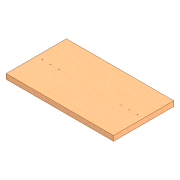
# Autodesk Inventor part: SGB-8-platform
Saved by Autodesk Inventor 2020 (Build 240168000, 168)
## iProperties
Created: 2021-06-24
Part Number: SGB-8-platform
Material: Generic
Document SubType Name: Modeling
Designer: Aidan Lee
Density: 1 g/cm^3
Appearance: Cherry - Natural Low Gloss
Author: Aidan Lee
Autodesk Inventor part; units mm, degrees
ref_plane "YZ Plane" through (0, 0, 0) normal (1, 0, 0) x (0, 1, 0)
ref_plane "XZ Plane" through (0, 0, 0) normal (0, 1, 0) x (-1, 0, 0)
ref_plane "XY Plane" through (0, 0, 0) normal (0, 0, 1) x (1, 0, 0)
sketch "Sketch2" plane through (0, 0, 0) normal (1, 0, 0) x (0, 1, 0)
  line L0 (0, 0) -> (18, 0)
  line L1 (18, 0) -> (18, 219)
  line L2 (18, 219) -> (0, 219)
  line L3 (0, 219) -> (0, 0)
  dimension "d2" = 18
  dimension "d3" = 219
  constraints: 8 end point, 2 parallel, 1 horizontal, 1 perpendicular
  measures "d2" distance of L0.start L0.end
  measures "d3" distance of L2.end L0.start
extrude "Extrusion1" add sketch "Sketch2" along normal blind 390.2
sketch "Sketch3" plane through (0, 18, 219) normal (0, 1, 0) x (1, 0, 0)
  line L0 (0, 118.5) -> (105, 118.5) construction
  line L1 (105, 118.5) -> (105, 100.5) construction
  line L2 (105, 100.5) -> (0, 100.5) construction
  line L3 (0, 100.5) -> (0, 118.5) construction
  circle A0 centre (22.5, 109.5) radius 1
  circle A1 centre (52.5, 109.5) radius 1
  circle A2 centre (82.5, 109.5) radius 1
  line L4 (0, 219) -> (0, 0) construction
  line L5 (0, 0) -> (390.2, 0) construction
  line L6 (195.1, 92.3564) -> (195.1, 74.6575) construction
  line L7 (390.2, 118.5) -> (285.2, 118.5) construction
  line L8 (285.2, 118.5) -> (285.2, 100.5) construction
  line L9 (285.2, 100.5) -> (390.2, 100.5) construction
  line L10 (390.2, 100.5) -> (390.2, 118.5) construction
  circle A3 centre (367.7, 109.5) radius 1
  circle A4 centre (337.7, 109.5) radius 1
  circle A5 centre (307.7, 109.5) radius 1
  line L11 (10, 90.5) -> (380.2, 90.5)
  line L12 (380.2, 90.5) -> (380.2, 10)
  line L13 (380.2, 10) -> (10, 10)
  line L14 (10, 10) -> (10, 90.5)
  line L15 (390.2, 219) -> (390.2, 0) projected
  point P0 (52.5, 100.5)
  point P1 (0, 109.5)
  point P2 (0, 109.5)
  point P3 (337.7, 100.5)
  point P4 (390.2, 109.5)
  dimension "d6" = 105
  dimension "d10" = 30
  dimension "d15" = 18
  dimension "screwholediameter" = 2
  dimension "d17" = 90.1
  dimension "d18" = 0
  dimension "d19" = 390.2
  dimension "d22" = 370.2
  dimension "d23" = 80.5
  dimension "d24" = 10
  dimension "d25" = 10
  dimension "d26" = 10
  dimension "d27" = 10
  constraints: 26 end point, 9 symmetric about line, 6 centre point, 4 parallel, 3 horizontal, 3 midpoint, 2 perpendicular, 1 coincident, 1 horizontal alignment, 1 vertical, 1 vertical alignment, 7 other
  measures "d6" distance of L1.end L2.end
  measures "d10" distance of A0.centre A1.centre
  measures "d15" distance of L2.end L0.start
  measures "screwholediameter" diameter of A0
  measures "d17" distance between parallel lines of L6 L1
  measures "d18" distance between parallel lines of L4 L3
  measures "d19" distance between parallel lines of L10 L3
  measures "d22" distance of L12.end L13.end
  measures "d23" distance of L13.end L11.start
  measures "d24" distance between parallel lines of L2 L11
  measures "d25" distance between parallel lines of L5 L13
  measures "d26" distance between parallel lines of L4 L14
  measures "d27" distance between parallel lines of L15 L12
extrude "Extrusion2" cut sketch "Sketch3" against normal through all contours A0 | A1 | A2 | A3 | A4 | A5
chamfer "Chamfer1" distance 1 angle 45 6 edges at (21.5, 0, 109.5) (51.5, 0, 109.5) (81.5, 0, 109.5) (306.7, 0, 109.5) (336.7, 0, 109.5) (366.7, 0, 109.5)
body "Solid1"
